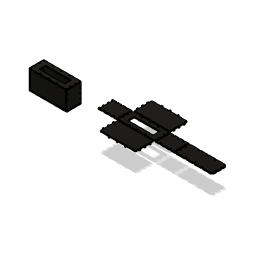
Case (Autodesk Fusion 360 design; units mm, degrees)
Autodesk Fusion 360 part; units mm, degrees
sketch "Sketch1" plane through (0, 0, 0) normal (0, 1, 0) x (1, 0, 0)
  line L0 (-40, -20) -> (150, -20)
  line L1 (150, -20) -> (150, 53.3)
  line L2 (150, 53.3) -> (-40, 53.3)
  line L3 (-40, 53.3) -> (-40, -20)
  line L4 (-40, 16.65) -> (-10, 16.65)
  line L5 (-10, -0.0029) -> (120, -0.0029)
  line L6 (120, 33.2971) -> (-10, 33.2971)
  line L7 (-10, 33.2971) -> (-10, -0.0029)
  line L8 (120, 33.2971) -> (120, -0.0029)
  dimension "d39" = 190
  dimension "d72" = 130
  dimension "d73" = 33.3
  constraint horizontal L0
  constraint vertical L1
  constraint horizontal L2
  constraint vertical L3
  constraint midpoint L3 L4.start
  constraint perpendicular L3 L4
  constraint vertical L7
  constraint perpendicular L5 L8
  measures "d39" distance of L1.end L2.end
  measures "d72" distance of L5.start L5.end
  measures "d73" distance of L5.start L6.end
extrude "Extrude6" add sketch "Sketch1" against normal blind 6 contours L0 L1 L2 L3 | L5 L6 L7 L8 makes body 1
sketch "Sketch3" plane through (-40, 0, 0) normal (-1, 0, 0) x (0, 0, 1)
  line L0 (20, 0) -> (-53.3, 0)
  line L1 (-53.3, 0) -> (-53.3, -6)
  line L2 (-53.3, -6) -> (20, -6)
  line L3 (20, -6) -> (20, 0)
  line L4 (-53.3, 0) -> (20, 0)
  line L5 (20, 0) -> (20, -100)
  line L6 (20, -100) -> (-53.3, -100)
  line L7 (-53.3, -100) -> (-53.3, 0)
  line L8 (20, 0) -> (14, 0)
  line L9 (14, 0) -> (14, -6)
  line L10 (20, -6) -> (20, 0)
  line L11 (14, -6) -> (-1, -6)
  line L12 (-7, -6) -> (-7, 0)
  line L13 (-7, 0) -> (-1, 0)
  line L14 (-1, 0) -> (-1, -6)
  line L15 (-53.3, 0) -> (-47.3, 0)
  line L16 (-47.3, 0) -> (-47.3, -6)
  line L17 (-53.3, -6) -> (-53.3, 0)
  line L18 (-47.3, -6) -> (-32.3, -6)
  line L19 (-26.3, -6) -> (-26.3, 0)
  line L20 (-26.3, 0) -> (-32.3, 0)
  line L21 (-32.3, 0) -> (-32.3, -6)
  dimension "d50" = 73.3
  dimension "d51" = 100
  dimension "d52" = 6
  dimension "d53" = 6
  dimension "d54" = 15
  dimension "d55" = 6
  dimension "d56" = 6
  dimension "d57" = 6
  dimension "d58" = 6
  dimension "d59" = 15
  dimension "d60" = 6
  dimension "d61" = 6
  constraint horizontal L4
  constraint vertical L5
  constraint horizontal L6
  constraint vertical L7
  constraint coincident L0.end L1.start
  constraint horizontal L8
  constraint vertical L9
  constraint vertical L10
  constraint coincident L0.start L3.end
  constraint perpendicular L9 L11
  constraint vertical L12
  constraint horizontal L13
  constraint vertical L14
  constraint horizontal L15
  constraint vertical L16
  constraint vertical L17
  constraint perpendicular L16 L18
  constraint vertical L19
  constraint horizontal L20
  constraint vertical L21
  measures "d50" distance of L0.end L0.start
  measures "d51" distance of L0.end L6.end
  measures "d52" distance of L0.start L8.end
  measures "d53" distance of L0.start L2.end
  measures "d54" distance of L9.end L11.end
  measures "d55" distance of L11.end L12.start
  measures "d56" distance of L11.end L13.end
  measures "d57" distance of L0.end L15.end
  measures "d58" distance of L0.end L1.end
  measures "d59" distance of L16.end L18.end
  measures "d60" distance of L18.end L19.start
  measures "d61" distance of L18.end L20.end
extrude "Extrude10" cut sketch "Sketch3" against normal blind 6 contours L0 L2 L3 L4 L5 L8 L9 L10 | L0 L2 L4 L12 L13 L14 | L0 L2 L4 L19 L20 L21 | L0 L1 L2 L4 L7 L15 L16 L17 bodies 1
extrude "Extrude7" cut sketch "Sketch3" against normal blind 6 contours L0 L1 L2 L4 L7 L15 L16 L17 bodies 1
extrude "Extrude8" cut sketch "Sketch3" against normal blind 6 contours L0 L2 L4 L19 L20 L21 bodies 1
extrude "Extrude9" cut sketch "Sketch3" against normal blind 6 contours L0 L2 L3 L4 L5 L8 L9 L10 | L0 L2 L4 L12 L13 L14 bodies 1
extrude "Extrude11" add sketch "Sketch3" against normal blind 6 separate body contours L0 L2 L3 L4 L5 L8 L9 L10 | L2 L5 L6 L7 L11 L18 | L0 L2 L4 L12 L13 L14 | L0 L2 L4 L19 L20 L21 | L0 L1 L2 L4 L7 L15 L16 L17 makes body 2
sketch "Sketch4" plane through (0, 0, 20) normal (0, 0, 1) x (1, 0, 0)
  line L0 (-40, 0) -> (-40, -100)
  line L1 (-40, -100) -> (-34, -100)
  line L2 (-34, -100) -> (-34, 0)
  line L3 (-34, 0) -> (-40, 0)
  line L4 (-40, 0) -> (150, 0)
  line L5 (150, 0) -> (150, -100)
  line L6 (150, -100) -> (-40, -100)
  line L7 (-40, -100) -> (-40, 0)
  line L8 (-40, 0) -> (-34, 0)
  line L9 (-34, 0) -> (-34, -6)
  line L10 (-34, -6) -> (-40, -6)
  line L11 (-40, -6) -> (-40, 0)
  line L12 (-40, -100) -> (-34, -100)
  line L13 (-34, -100) -> (-34, -94)
  line L14 (-34, -94) -> (-40, -94)
  line L15 (-40, -94) -> (-40, -100)
  line L16 (-40, -94) -> (-40, -79)
  line L17 (-40, -79) -> (-34, -79)
  line L18 (-34, -79) -> (-34, -73)
  line L19 (-34, -73) -> (-40, -73)
  line L20 (-40, -73) -> (-40, -79)
  line L21 (-40, -6) -> (-40, -21)
  line L22 (-40, -21) -> (-34, -21)
  line L23 (-34, -21) -> (-34, -27)
  line L24 (-34, -27) -> (-40, -27)
  line L25 (-40, -27) -> (-40, -21)
  line L26 (-40, -27) -> (-40, -47)
  line L27 (-40, -47) -> (-34, -47)
  line L28 (-34, -47) -> (-34, -53)
  line L29 (-34, -53) -> (-40, -53)
  line L30 (-40, -53) -> (-40, -47)
  line L31 (52, 0) -> (58, 0)
  line L32 (58, 0) -> (58, -6)
  line L33 (58, -6) -> (52, -6)
  line L34 (52, -6) -> (52, 0)
  line L35 (52, 0) -> (17, 0)
  line L36 (58, 0) -> (93, 0)
  line L37 (17, 0) -> (11, 0)
  line L38 (11, 0) -> (11, -6)
  line L39 (11, -6) -> (17, -6)
  line L40 (17, -6) -> (17, 0)
  line L41 (93, 0) -> (99, 0)
  line L42 (99, 0) -> (99, -6)
  line L43 (99, -6) -> (93, -6)
  line L44 (93, -6) -> (93, 0)
  line L45 (144, -27) -> (144, -21)
  line L46 (150, -27) -> (144, -27)
  line L47 (150, -53) -> (144, -53)
  line L48 (144, -73) -> (144, -79)
  line L49 (150, -79) -> (150, -73)
  line L50 (150, -73) -> (144, -73)
  line L51 (144, -79) -> (150, -79)
  line L52 (144, -47) -> (150, -47)
  line L53 (150, -47) -> (150, -53)
  line L54 (144, -27) -> (144, -47)
  line L55 (144, -53) -> (144, -47)
  line L56 (150, -21) -> (150, -27)
  line L57 (144, -21) -> (150, -21)
  line L58 (-34, -6) -> (150, -6)
  line L59 (150, 0) -> (144, 0)
  line L60 (144, 0) -> (144, -6)
  line L61 (144, -6) -> (150, -6)
  line L62 (150, -6) -> (150, 0)
  line L63 (144, -6) -> (144, -100)
  dimension "d76" = 6
  dimension "d77" = 6
  dimension "d78" = 6
  dimension "d79" = 6
  dimension "d80" = 15
  dimension "d81" = 6
  dimension "d82" = 6
  dimension "d83" = 15
  dimension "d84" = 6
  dimension "d85" = 6
  dimension "d86" = 20
  dimension "d87" = 6
  dimension "d88" = 6
  dimension "d93" = 190
  dimension "d95" = 6
  dimension "d96" = 6
  dimension "d97" = 35
  dimension "d98" = 35
  dimension "d99" = 6
  dimension "d100" = 6
  dimension "d101" = 6
  dimension "d102" = 6
  dimension "d103" = 6
  dimension "d104" = 6
  dimension "d105" = 6
  dimension "d106" = 6
  dimension "d107" = 20
  dimension "d108" = 6
  dimension "d109" = 6
  dimension "d122" = 6
  dimension "d123" = 6
  dimension "d124" = 94
  constraint horizontal L4
  constraint vertical L5
  constraint horizontal L6
  constraint vertical L7
  constraint coincident L0.start L3.end
  constraint horizontal L8
  constraint vertical L9
  constraint horizontal L10
  constraint vertical L11
  constraint horizontal L12
  constraint vertical L13
  constraint horizontal L14
  constraint vertical L15
  constraint coincident L0.end L1.start
  constraint perpendicular L14 L16
  constraint horizontal L17
  constraint vertical L18
  constraint horizontal L19
  constraint vertical L20
  constraint perpendicular L10 L21
  constraint horizontal L22
  constraint vertical L23
  constraint horizontal L24
  constraint vertical L25
  constraint perpendicular L24 L26
  constraint horizontal L27
  constraint vertical L28
  constraint horizontal L29
  constraint vertical L30
  constraint horizontal L31
  constraint vertical L32
  constraint horizontal L33
  constraint vertical L34
  constraint perpendicular L34 L35
  constraint perpendicular L32 L36
  constraint horizontal L37
  constraint vertical L38
  constraint horizontal L39
  constraint vertical L40
  constraint horizontal L41
  constraint vertical L42
  constraint horizontal L43
  constraint vertical L44
  constraint horizontal L51
  constraint vertical L49
  constraint horizontal L50
  constraint vertical L48
  constraint horizontal L57
  constraint vertical L56
  constraint horizontal L46
  constraint vertical L45
  constraint perpendicular L46 L54
  constraint horizontal L52
  constraint vertical L53
  constraint horizontal L47
  constraint vertical L55
  constraint coincident L5 L58.end
  constraint perpendicular L5 L58
  constraint horizontal L59
  constraint vertical L60
  constraint horizontal L61
  constraint vertical L62
  constraint perpendicular L46 L63
  measures "d76" distance of L0.start L2.end
  measures "d77" distance of L0.start L10.end
  measures "d78" distance of L0.end L1.end
  measures "d79" distance of L0.end L14.end
  measures "d80" distance of L14.end L16.end
  measures "d81" distance of L16.end L17.end
  measures "d82" distance of L16.end L19.end
  measures "d83" distance of L10.end L21.end
  measures "d84" distance of L21.end L22.end
  measures "d85" distance of L21.end L24.end
  measures "d86" distance of L24.end L26.end
  measures "d87" distance of L26.end L27.end
  measures "d88" distance of L26.end L29.end
  measures "d93" distance of L0.start L4.end
  measures "d95" distance of L31.start L31.end
  measures "d96" distance of L31.start L33.end
  measures "d97" distance of L31.start L35.end
  measures "d98" distance of L31.end L36.end
  measures "d99" distance of L35.end L37.end
  measures "d100" distance of L35.end L39.end
  measures "d101" distance of L36.end L41.end
  measures "d102" distance of L36.end L43.end
  measures "d103" distance of L49.start L48.end
  measures "d104" distance of L48.end L48.start
  measures "d105" distance of L56.start L45.end
  measures "d106" distance of L45.start L45.end
  measures "d107" distance of L45.start L52.start
  measures "d108" distance of L52.end L52.start
  measures "d109" distance of L47.end L52.start
  measures "d122" distance of L4.end L59.end
  measures "d123" distance of L4.end L58.end
  measures "d124" distance of L60.end L63.end
extrude "Extrude13" cut sketch "Sketch4" against normal blind 6 contours L0 L2 L7 L22 L23 L24 L25 | L0 L2 L7 L27 L28 L29 L30 | L0 L2 L7 L17 L18 L19 L20 bodies 2
extrude "Extrude12" cut sketch "Sketch1" against normal blind 6 contours L5 L6 L7 L8 bodies 1
copy_body "CopyPasteBodies1" bodies 2 makes body 3
move_body "Move1" bodies 3 to x (1, 0, 0) y (0, 1, 0) z (0, 0, 1) at (184, 0, 0)
sketch "Sketch5" plane through (0, 0, 0) normal (0, 1, 0) x (1, 0, 0)
  line L0 (150, 53.3) -> (144, 53.3)
  line L1 (144, 53.3) -> (144, 47.3)
  line L2 (144, 47.3) -> (150, 47.3)
  line L3 (150, 47.3) -> (150, 53.3)
  line L4 (150, 32.3) -> (144, 32.3)
  line L5 (144, 32.3) -> (144, 26.3)
  line L6 (144, 26.3) -> (150, 26.3)
  line L7 (150, 26.3) -> (150, 32.3)
  line L8 (150, 1) -> (144, 1)
  line L9 (144, 1) -> (144, 7)
  line L10 (144, 7) -> (150, 7)
  line L11 (150, 7) -> (150, 1)
  line L12 (150, -20) -> (144, -20)
  line L13 (144, -20) -> (144, -14)
  line L14 (144, -14) -> (150, -14)
  line L15 (150, -14) -> (150, -20)
  dimension "d110" = 6
  dimension "d111" = 6
  dimension "d112" = 6
  dimension "d113" = 6
  dimension "d114" = 6
  dimension "d115" = 6
  dimension "d116" = 6
  dimension "d117" = 6
  constraint horizontal L0
  constraint vertical L1
  constraint horizontal L2
  constraint vertical L3
  constraint horizontal L4
  constraint vertical L5
  constraint horizontal L6
  constraint vertical L7
  constraint horizontal L8
  constraint vertical L9
  constraint horizontal L10
  constraint vertical L11
  constraint horizontal L12
  constraint vertical L13
  constraint horizontal L14
  constraint vertical L15
  measures "d110" distance of L0.start L0.end
  measures "d111" distance of L0.start L2.end
  measures "d112" distance of L4.start L4.end
  measures "d113" distance of L4.start L6.end
  measures "d114" distance of L8.start L8.end
  measures "d115" distance of L8.start L10.end
  measures "d116" distance of L12.start L12.end
  measures "d117" distance of L12.start L14.end
extrude "Extrude15" cut sketch "Sketch5" against normal blind 6 bodies 1
extrude "Extrude16" cut sketch "Sketch4" against normal blind 6 contours L4 L37 L38 L39 L40 L58 | L4 L31 L32 L33 L34 L58 | L4 L41 L42 L43 L44 L58 bodies 1
extrude "Extrude17" add sketch "Sketch4" against normal blind 6 separate body contours L0 L2 L7 L22 L23 L24 L25 | L2 L6 L13 L18 L23 L28 L33 L39 L43 L45 L48 L54 L55 L58 L63 | L4 L37 L38 L39 L40 L58 | L0 L2 L7 L27 L28 L29 L30 | L4 L31 L32 L33 L34 L58 | L0 L2 L7 L17 L18 L19 L20 | L4 L41 L42 L43 L44 L58 | L5 L45 L46 L56 L57 L63 | L5 L48 L49 L50 L51 L63 | L5 L47 L52 L53 L55 L63 makes body 4
sketch "fundo" plane through (0, 0, -53.3) normal (0, 0, -1) x (-1, 0, 0)
  line L0 (40, -100) -> (40, 0)
  line L1 (40, 0) -> (34, 0)
  line L2 (34, 0) -> (34, -100)
  line L3 (34, -100) -> (40, -100)
  line L4 (40, 0) -> (-150, 0)
  line L5 (-150, 0) -> (-150, -100)
  line L6 (-150, -100) -> (40, -100)
  line L7 (40, -100) -> (40, 0)
  line L8 (-150, 0) -> (-144, 0)
  line L9 (-144, 0) -> (-144, -6)
  line L10 (-144, -6) -> (-150, -6)
  line L11 (-150, -6) -> (-150, 0)
  line L12 (-55, 0) -> (-58, 0)
  line L13 (-58, 0) -> (-52, 0)
  line L14 (-52, 0) -> (-52, -6)
  line L15 (-52, -6) -> (-58, -6)
  line L16 (-58, -6) -> (-58, 0)
  line L17 (-58, 0) -> (-93, 0)
  line L18 (-93, 0) -> (-99, 0)
  line L19 (-99, 0) -> (-99, -6)
  line L20 (-99, -6) -> (-93, -6)
  line L21 (-93, -6) -> (-93, 0)
  line L22 (-52, 0) -> (-17, 0)
  line L23 (-17, 0) -> (-11, 0)
  line L24 (-11, 0) -> (-11, -6)
  line L25 (-11, -6) -> (-17, -6)
  line L26 (-17, -6) -> (-17, 0)
  line L27 (-150, 0) -> (-150, -21)
  line L28 (40, 0) -> (40, -21)
  line L29 (-150, -21) -> (-144, -21)
  line L30 (-144, -21) -> (-144, -27)
  line L31 (-144, -27) -> (-150, -27)
  line L32 (-150, -27) -> (-150, -21)
  line L33 (40, -21) -> (34, -21)
  line L34 (34, -21) -> (34, -27)
  line L35 (34, -27) -> (40, -27)
  line L36 (40, -27) -> (40, -21)
  line L37 (-144, -27) -> (-144, -47)
  line L38 (-144, -47) -> (-150, -47)
  line L39 (-150, -47) -> (-150, -53)
  line L40 (-150, -53) -> (-144, -53)
  line L41 (-144, -53) -> (-144, -47)
  line L42 (-144, -53) -> (-144, -73)
  line L43 (-144, -73) -> (-150, -73)
  line L44 (-150, -73) -> (-150, -79)
  line L45 (-150, -79) -> (-144, -79)
  line L46 (-144, -79) -> (-144, -73)
  line L47 (40, -27) -> (40, -47)
  line L48 (40, -47) -> (34, -47)
  line L49 (34, -47) -> (34, -53)
  line L50 (34, -53) -> (40, -53)
  line L51 (40, -53) -> (40, -47)
  line L52 (40, -53) -> (40, -73)
  line L53 (40, -73) -> (34, -73)
  line L54 (34, -73) -> (34, -79)
  line L55 (34, -79) -> (40, -79)
  line L56 (40, -79) -> (40, -73)
  line L57 (34, 0) -> (34, -100)
  line L58 (-144, 0) -> (-144, -100)
  line L59 (-150, -6) -> (40, -6)
  dimension "d127" = 6
  dimension "d128" = 6
  dimension "d129" = 3
  dimension "d130" = 6
  dimension "d131" = 6
  dimension "d132" = 35
  dimension "d133" = 6
  dimension "d134" = 6
  dimension "d135" = 35
  dimension "d136" = 6
  dimension "d137" = 6
  dimension "d140" = 21
  dimension "d141" = 21
  dimension "d142" = 6
  dimension "d143" = 6
  dimension "d144" = 6
  dimension "d145" = 6
  dimension "d146" = 20
  dimension "d147" = 6
  dimension "d148" = 20
  dimension "d149" = 6
  dimension "d150" = 6
  dimension "d151" = 20
  dimension "d152" = 6
  dimension "d153" = 6
  dimension "d154" = 20
  dimension "d155" = 6
  dimension "d156" = 6
  dimension "d159" = 190
  constraint horizontal L4
  constraint vertical L5
  constraint horizontal L6
  constraint vertical L7
  constraint coincident L0.end L1.start
  constraint horizontal L8
  constraint vertical L9
  constraint horizontal L10
  constraint vertical L11
  constraint midpoint L4 L12.start
  constraint parallel L4 L12
  constraint horizontal L13
  constraint vertical L14
  constraint horizontal L15
  constraint vertical L16
  constraint perpendicular L16 L17
  constraint horizontal L18
  constraint vertical L19
  constraint horizontal L20
  constraint vertical L21
  constraint perpendicular L14 L22
  constraint horizontal L23
  constraint vertical L24
  constraint horizontal L25
  constraint vertical L26
  constraint perpendicular L4 L27
  constraint perpendicular L4 L28
  constraint horizontal L29
  constraint vertical L30
  constraint horizontal L31
  constraint vertical L32
  constraint horizontal L33
  constraint vertical L34
  constraint horizontal L35
  constraint vertical L36
  constraint perpendicular L31 L37
  constraint horizontal L38
  constraint vertical L39
  constraint horizontal L40
  constraint vertical L41
  constraint perpendicular L40 L42
  constraint horizontal L43
  constraint vertical L44
  constraint horizontal L45
  constraint vertical L46
  constraint perpendicular L35 L47
  constraint horizontal L48
  constraint vertical L49
  constraint horizontal L50
  constraint vertical L51
  constraint perpendicular L50 L52
  constraint horizontal L53
  constraint vertical L54
  constraint horizontal L55
  constraint vertical L56
  constraint coincident L1.end L2.start
  constraint coincident L2.end L3.start
  constraint coincident L6 L58.end
  constraint perpendicular L6 L58
  constraint horizontal L59
  measures "d127" distance of L4.end L8.end
  measures "d128" distance of L4.end L10.end
  measures "d129" distance of L12.start L12.end
  measures "d130" distance of L12.end L13.end
  measures "d131" distance of L12.end L15.end
  measures "d132" distance of L12.end L17.end
  measures "d133" distance of L17.end L18.end
  measures "d134" distance of L17.end L20.end
  measures "d135" distance of L13.end L22.end
  measures "d136" distance of L22.end L23.end
  measures "d137" distance of L22.end L25.end
  measures "d140" distance of L4.end L27.end
  measures "d141" distance of L0.end L28.end
  measures "d142" distance of L27.end L29.end
  measures "d143" distance of L27.end L31.end
  measures "d144" distance of L28.end L33.end
  measures "d145" distance of L28.end L35.end
  measures "d146" distance of L30.end L37.end
  measures "d147" distance of L37.end L40.end
  measures "d148" distance of L40.end L42.end
  measures "d149" distance of L42.end L43.end
  measures "d150" distance of L42.end L45.end
  measures "d151" distance of L35.end L47.end
  measures "d152" distance of L47.end L48.end
  measures "d153" distance of L47.end L50.end
  measures "d154" distance of L50.end L52.end
  measures "d155" distance of L52.end L53.end
  measures "d156" distance of L52.end L55.end
  measures "d159" distance of L10.end L59.end
extrude "Extrude18" cut sketch "fundo" against normal blind 6 contours L4 L23 L24 L25 L26 L59 | L4 L18 L19 L20 L21 L59 | L4 L12 L13 L14 L15 L16 L59 bodies 1
extrude "Extrude19" cut sketch "fundo" against normal blind 6 contours L0 L2 L7 L53 L54 L55 L56 L57 | L0 L2 L7 L48 L49 L50 L51 L57 | L5 L43 L44 L45 L46 L58 | L0 L2 L7 L33 L34 L35 L36 L57 | L5 L38 L39 L40 L41 L58 | L5 L29 L30 L31 L32 L58 bodies 2 3
extrude "Extrude20" add sketch "fundo" against normal blind 6 separate body contours L0 L2 L7 L53 L54 L55 L56 L57 | L2 L6 L15 L20 L25 L30 L34 L37 L41 L42 L46 L49 L54 L57 L58 L59 | L0 L2 L7 L48 L49 L50 L51 L57 | L5 L43 L44 L45 L46 L58 | L0 L2 L7 L33 L34 L35 L36 L57 | L5 L38 L39 L40 L41 L58 | L5 L29 L30 L31 L32 L58 | L4 L23 L24 L25 L26 L59 | L4 L18 L19 L20 L21 L59 | L4 L12 L13 L14 L15 L16 L59 makes body 5
sketch "Sketch7" plane through (0, -100, 0) normal (0, -1, 0) x (1, 0, 0)
  line L0 (-34, -53.3) -> (144, -53.3)
  line L1 (144, -53.3) -> (144, -47.3)
  line L2 (144, -47.3) -> (-34, -47.3)
  line L3 (-34, -47.3) -> (-34, -53.3)
  line L4 (-40, -53.3) -> (150, -53.3)
  line L5 (150, -53.3) -> (150, 20)
  line L6 (150, 20) -> (-40, 20)
  line L7 (-40, 20) -> (-40, -53.3)
  line L8 (144, -53.3) -> (150, -53.3)
  line L9 (150, -53.3) -> (150, 20)
  line L10 (150, 20) -> (144, 20)
  line L11 (144, 20) -> (144, -53.3)
  line L12 (-34, -53.3) -> (-40, -53.3)
  line L13 (-40, -53.3) -> (-40, 20)
  line L14 (-40, 20) -> (-34, 20)
  line L15 (-34, 20) -> (-34, -53.3)
  line L16 (-40, 20) -> (150, 20)
  line L17 (150, 20) -> (150, 14)
  line L18 (150, 14) -> (-40, 14)
  line L19 (-40, 14) -> (-40, 20)
  line L20 (55, 14) -> (52.5, 14)
  line L21 (52.5, 14) -> (57.5, 14)
  arc A0 (52.5, 14) -> (57.5, 14) centre (55, 12.125) ccw
  line L22 (-40, 14) -> (-40, -1)
  line L23 (-40, -1) -> (-34, -1)
  line L24 (-34, -1) -> (-34, -7)
  line L25 (-34, -7) -> (-40, -7)
  line L26 (-40, -7) -> (-40, -1)
  line L27 (-40, -7) -> (-40, -26.3)
  line L28 (-40, -26.3) -> (-34, -26.3)
  line L29 (-34, -26.3) -> (-34, -32.3)
  line L30 (-34, -32.3) -> (-40, -32.3)
  line L31 (-40, -32.3) -> (-40, -26.3)
  line L32 (-40, -53.3) -> (-34, -53.3)
  line L33 (-34, -53.3) -> (-34, -47.3)
  line L34 (-34, -47.3) -> (-40, -47.3)
  line L35 (-40, -47.3) -> (-40, -53.3)
  line L36 (150, -47.3) -> (150, -53.3)
  line L37 (150, -7) -> (144, -7)
  line L38 (144, -1) -> (150, -1)
  line L39 (144, -26.3) -> (150, -26.3)
  line L40 (144, -47.3) -> (144, -53.3)
  line L41 (144, -53.3) -> (144, 20)
  line L42 (144, 14) -> (144, -1)
  line L43 (144, 14) -> (144, 20)
  line L44 (150, -32.3) -> (144, -32.3)
  line L45 (150, -47.3) -> (144, -47.3)
  line L46 (144, -53.3) -> (150, -53.3)
  line L47 (150, -53.3) -> (150, -47.3)
  line L48 (144, 20) -> (150, 20)
  line L49 (150, -1) -> (150, -7)
  line L50 (144, -7) -> (144, -1)
  line L51 (150, -53.3) -> (144, -53.3)
  line L52 (150, -26.3) -> (150, -32.3)
  line L53 (144, -7) -> (144, -26.3)
  line L54 (150, 20) -> (150, -53.3)
  line L55 (144, 20) -> (144, -53.3)
  line L56 (144, -32.3) -> (144, -26.3)
  line L57 (-34, 20) -> (11, 20)
  line L58 (11, 20) -> (11, 14)
  line L59 (11, 14) -> (-34, 14)
  line L60 (-34, 14) -> (-34, 20)
  line L61 (11, 20) -> (17, 20)
  line L62 (17, 20) -> (17, 14)
  line L63 (17, 14) -> (11, 14)
  line L64 (11, 14) -> (11, 20)
  line L65 (17, 20) -> (52, 20)
  line L66 (52, 20) -> (52, 14)
  line L67 (52, 14) -> (17, 14)
  line L68 (17, 14) -> (17, 20)
  line L69 (52, 20) -> (58, 20)
  line L70 (58, 20) -> (58, 14)
  line L71 (58, 14) -> (52, 14)
  line L72 (52, 14) -> (52, 20)
  line L73 (58, 20) -> (93, 20)
  line L74 (93, 20) -> (93, 14)
  line L75 (93, 14) -> (58, 14)
  line L76 (58, 14) -> (58, 20)
  line L77 (93, 20) -> (99, 20)
  line L78 (99, 20) -> (99, 14)
  line L79 (99, 14) -> (93, 14)
  line L80 (93, 14) -> (93, 20)
  line L81 (144, -53.3) -> (99, -53.3)
  line L82 (99, -53.3) -> (93, -53.3)
  line L83 (93, -53.3) -> (93, -47.3)
  line L84 (93, -47.3) -> (99, -47.3)
  line L85 (99, -47.3) -> (99, -53.3)
  line L86 (93, -53.3) -> (58, -53.3)
  line L87 (58, -53.3) -> (58, -47.3)
  line L88 (58, -47.3) -> (93, -47.3)
  line L89 (93, -47.3) -> (93, -53.3)
  line L90 (58, -53.3) -> (52, -53.3)
  line L91 (52, -53.3) -> (52, -47.3)
  line L92 (52, -47.3) -> (58, -47.3)
  line L93 (58, -47.3) -> (58, -53.3)
  line L94 (52, -53.3) -> (17, -53.3)
  line L95 (17, -53.3) -> (17, -47.3)
  line L96 (17, -47.3) -> (52, -47.3)
  line L97 (52, -47.3) -> (52, -53.3)
  line L98 (17, -53.3) -> (11, -53.3)
  line L99 (11, -53.3) -> (11, -47.3)
  line L100 (11, -47.3) -> (17, -47.3)
  line L101 (17, -47.3) -> (17, -53.3)
  dimension "d162" = 190
  dimension "d163" = 73.3
  dimension "d164" = 6
  dimension "d169" = 5
  dimension "d171" = 3.125
  dimension "d172" = 15
  dimension "d173" = 6
  dimension "d174" = 6
  dimension "d175" = 19.3
  dimension "d176" = 6
  dimension "d177" = 6
  dimension "d178" = 6
  dimension "d179" = 6
  dimension "d182" = 73.3
  dimension "d183" = 6
  dimension "d184" = 15
  dimension "d185" = 6
  dimension "d186" = 6
  dimension "d187" = 19.3
  dimension "d188" = 6
  dimension "d189" = 6
  dimension "d190" = 6
  dimension "d191" = 6
  dimension "d194" = 45
  dimension "d195" = 6
  dimension "d196" = 6
  dimension "d197" = 6
  dimension "d198" = 35
  dimension "d199" = 6
  dimension "d200" = 6
  dimension "d201" = 6
  dimension "d202" = 35
  dimension "d203" = 6
  dimension "d204" = 6
  dimension "d205" = 6
  dimension "d208" = 45
  dimension "d209" = 6
  dimension "d210" = 6
  dimension "d211" = 35
  dimension "d212" = 6
  dimension "d213" = 6
  dimension "d214" = 6
  dimension "d215" = 35
  dimension "d216" = 6
  dimension "d217" = 6
  dimension "d218" = 6
  constraint horizontal L4
  constraint vertical L5
  constraint horizontal L6
  constraint vertical L7
  constraint horizontal L8
  constraint vertical L9
  constraint horizontal L10
  constraint vertical L11
  constraint coincident L0.end L1.start
  constraint horizontal L12
  constraint vertical L13
  constraint horizontal L14
  constraint vertical L15
  constraint coincident L0.start L3.end
  constraint horizontal L16
  constraint vertical L17
  constraint horizontal L18
  constraint vertical L19
  constraint symmetric L18 L20.end L21.start
  constraint symmetric L18 L21.end A0.end
  constraint perpendicular L18 L22
  constraint horizontal L23
  constraint vertical L24
  constraint horizontal L25
  constraint vertical L26
  constraint perpendicular L25 L27
  constraint horizontal L28
  constraint vertical L29
  constraint horizontal L30
  constraint vertical L31
  constraint horizontal L32
  constraint vertical L33
  constraint horizontal L34
  constraint vertical L35
  constraint vertical L55
  constraint horizontal L51
  constraint vertical L41
  constraint horizontal L48
  constraint vertical L54
  constraint coincident L4.end L5.start
  constraint vertical L43
  constraint horizontal L38
  constraint vertical L49
  constraint horizontal L37
  constraint vertical L50
  constraint perpendicular L37 L53
  constraint horizontal L39
  constraint vertical L52
  constraint horizontal L44
  constraint vertical L56
  constraint horizontal L46
  constraint vertical L47
  constraint horizontal L45
  constraint vertical L40
  constraint horizontal L57
  constraint vertical L58
  constraint horizontal L59
  constraint vertical L60
  constraint horizontal L61
  constraint vertical L62
  constraint horizontal L63
  constraint vertical L64
  constraint horizontal L65
  constraint vertical L66
  constraint horizontal L67
  constraint vertical L68
  constraint horizontal L69
  constraint vertical L70
  constraint horizontal L71
  constraint vertical L72
  constraint horizontal L73
  constraint vertical L74
  constraint horizontal L75
  constraint vertical L76
  constraint horizontal L77
  constraint vertical L78
  constraint horizontal L79
  constraint vertical L80
  constraint perpendicular L11 L81
  constraint horizontal L82
  constraint vertical L83
  constraint horizontal L84
  constraint vertical L85
  constraint horizontal L86
  constraint vertical L87
  constraint horizontal L88
  constraint vertical L89
  constraint horizontal L90
  constraint vertical L91
  constraint horizontal L92
  constraint vertical L93
  constraint horizontal L94
  constraint vertical L95
  constraint horizontal L96
  constraint vertical L97
  constraint horizontal L98
  constraint vertical L99
  constraint horizontal L100
  constraint vertical L101
  measures "d162" distance of L4.start L4.end
  measures "d163" distance of L4.start L6.end
  measures "d164" distance of L6.end L18.end
  measures "d169" distance of L20.end L21.end
  measures "d171" radius of A0
  measures "d172" distance of L18.end L22.end
  measures "d173" distance of L22.end L23.end
  measures "d174" distance of L22.end L25.end
  measures "d175" distance of L25.end L27.end
  measures "d176" distance of L27.end L28.end
  measures "d177" distance of L27.end L30.end
  measures "d178" distance of L4.start L0.start
  measures "d179" distance of L4.start L34.end
  measures "d182" distance of L0.end L10.end
  measures "d183" distance of L10.end L42.start
  measures "d184" distance of L38.start L42.start
  measures "d185" distance of L38.start L38.end
  measures "d186" distance of L38.start L37.end
  measures "d187" distance of L39.start L37.end
  measures "d188" distance of L39.end L39.start
  measures "d189" distance of L39.start L44.end
  measures "d190" distance of L4.end L0.end
  measures "d191" distance of L1.end L0.end
  measures "d194" distance of L14.end L57.end
  measures "d195" distance of L14.end L59.end
  measures "d196" distance of L57.end L61.end
  measures "d197" distance of L57.end L58.end
  measures "d198" distance of L61.end L65.end
  measures "d199" distance of L61.end L62.end
  measures "d200" distance of L65.end L69.end
  measures "d201" distance of L65.end L66.end
  measures "d202" distance of L69.end L73.end
  measures "d203" distance of L69.end L70.end
  measures "d204" distance of L73.end L77.end
  measures "d205" distance of L73.end L74.end
  measures "d208" distance of L0.end L81.end
  measures "d209" distance of L81.end L82.end
  measures "d210" distance of L81.end L84.end
  measures "d211" distance of L82.end L86.end
  measures "d212" distance of L82.end L83.end
  measures "d213" distance of L86.end L90.end
  measures "d214" distance of L86.end L87.end
  measures "d215" distance of L90.end L94.end
  measures "d216" distance of L90.end L91.end
  measures "d217" distance of L94.end L98.end
  measures "d218" distance of L94.end L95.end
extrude "Extrude23" cut sketch "Sketch7" against normal blind 6 contours L6 L15 L16 L18 L57 L58 L59 L60 L64 | L6 L16 L18 L62 L65 L66 L67 L68 L72 | L6 L16 L18 L70 L73 L74 L75 L76 L80 | L6 L11 L16 L18 L41 L43 L55 L78 bodies 4
extrude "Extrude22" cut sketch "Sketch7" against normal blind 6 contours L5 L9 L11 L41 L44 L45 L54 L55 | L5 L9 L11 L37 L39 L41 L53 L54 L55 | L5 L9 L11 L18 L38 L41 L42 L54 L55 bodies 3
extrude "Extrude21" cut sketch "Sketch7" against normal blind 6 contours L7 L13 L15 L30 L34 | L7 L13 L15 L25 L27 L28 | L7 L13 L15 L18 L22 L23 bodies 2
extrude "Extrude24" cut sketch "Sketch7" against normal blind 6 contours L0 L2 L3 L4 L15 L33 L99 | L0 L2 L4 L91 L94 L95 L96 L97 L101 | L0 L2 L4 L83 L86 L87 L88 L89 L93 | L0 L1 L2 L4 L11 L40 L41 L55 L81 L85 bodies 5
extrude "Extrude25" add sketch "Sketch7" against normal blind 6 separate body contours L0 L2 L3 L4 L15 L33 L99 | L2 L11 L15 L18 A0 L24 L29 L41 L42 L50 L53 L55 L56 L59 L63 L67 L71 L75 L79 L84 L88 L92 L96 L100 | L7 L13 L15 L30 L34 | L0 L2 L4 L91 L94 L95 L96 L97 L101 | L7 L13 L15 L25 L27 L28 | L0 L2 L4 L83 L86 L87 L88 L89 L93 | L7 L13 L15 L18 L22 L23 | L0 L1 L2 L4 L11 L40 L41 L55 L81 L85 | L6 L15 L16 L18 L57 L58 L59 L60 L64 | L5 L9 L11 L41 L44 L45 L54 L55 | L6 L16 L18 L62 L65 L66 L67 L68 L72 | L5 L9 L11 L37 L39 L41 L53 L54 L55 | L6 L16 L18 L70 L73 L74 L75 L76 L80 | L5 L9 L11 L18 L38 L41 L42 L54 L55 | L6 L11 L16 L18 L41 L43 L55 L78 makes body 6
copy_body "CopyPasteBodies2" bodies 1 6 2 5 3 4 makes body 7 makes body 8 makes body 9 makes body 10 makes body 11 makes body 12
move_body "Move2" bodies 7 8 9 10 11 12 to x (1, 0, 0) y (0, 1, 0) z (0, 0, 1) at (250, 0, 0)
move_body "Move3" bodies 10 to x (1, 0, 0) y (0, 0, 1) z (0, -1, 0) at (0, -53.3, -53.3)
move_body "Move4" bodies 12 to x (1, 0, 0) y (0, 0, -1) z (0, 1, 0) at (0, -20, 20)
move_body "Move5" bodies 12 10 7 9 8 11 to x (1, 0, 0) y (0, 1, 0) z (0, 0, 1) at (200, 0, 0)
move_body "Move6" bodies 9 to x (0, -1, 0) y (1, 0, 0) z (0, 0, 1) at (410, 410, 0)
move_body "Move7" bodies 8 to x (0, 1, 0) y (-1, 0, 0) z (0, 0, 1) at (500, -700, 0)
move_body "Move8" bodies 8 11 to x (0, 1, 0) y (-1, 0, 0) z (0, 0, 1) at (600, -600, 0)
sketch "cima plano" plane through (0, 0, 0) normal (0, 1, 0) x (-1, 0, 0)
  line L0 (-502, -153.3) -> (-502, -147.3)
  line L1 (-502, -147.3) -> (-467, -147.3)
  line L2 (-467, -147.3) -> (-467, -153.3)
  line L3 (-467, -153.3) -> (-461, -153.3)
  line L4 (-461, -153.3) -> (-461, -147.3)
  line L5 (-461, -147.3) -> (-416, -147.3)
  line L6 (-416, -147.3) -> (-416, -132.3)
  line L7 (-416, -132.3) -> (-410, -132.3)
  line L8 (-410, -132.3) -> (-410, -126.3)
  line L9 (-410, -126.3) -> (-416, -126.3)
  line L10 (-416, -126.3) -> (-416, -106.3)
  line L11 (-416, -106.3) -> (-410, -106.3)
  line L12 (-410, -106.3) -> (-410, -100.3)
  line L13 (-410, -100.3) -> (-416, -100.3)
  line L14 (-416, -100.3) -> (-416, -80.3)
  line L15 (-416, -80.3) -> (-410, -80.3)
  line L16 (-410, -80.3) -> (-410, -74.3)
  line L17 (-410, -74.3) -> (-416, -74.3)
  line L18 (-416, -74.3) -> (-416, -59.3)
  line L19 (-416, -59.3) -> (-461, -59.3)
  line L20 (-461, -59.3) -> (-461, -53.3)
  line L21 (-461, -53.3) -> (-467, -53.3)
  line L22 (-467, -53.3) -> (-467, -59.3)
  line L23 (-467, -59.3) -> (-502, -59.3)
  line L24 (-502, -59.3) -> (-502, -53.3)
  line L25 (-502, -53.3) -> (-508, -53.3)
  line L26 (-508, -53.3) -> (-508, -59.3)
  line L27 (-508, -59.3) -> (-543, -59.3)
  line L28 (-543, -59.3) -> (-543, -53.3)
  line L29 (-543, -53.3) -> (-549, -53.3)
  line L30 (-549, -53.3) -> (-549, -59.3)
  line L31 (-549, -59.3) -> (-594, -59.3)
  line L32 (-594, -59.3) -> (-594, -74.3)
  line L33 (-594, -74.3) -> (-600, -74.3)
  line L34 (-600, -74.3) -> (-600, -80.3)
  line L35 (-600, -80.3) -> (-594, -80.3)
  line L36 (-594, -80.3) -> (-594, -100.3)
  line L37 (-594, -100.3) -> (-600, -100.3)
  line L38 (-600, -100.3) -> (-600, -106.3)
  line L39 (-600, -106.3) -> (-594, -106.3)
  line L40 (-594, -106.3) -> (-594, -126.3)
  line L41 (-594, -126.3) -> (-600, -126.3)
  line L42 (-600, -126.3) -> (-600, -132.3)
  line L43 (-600, -132.3) -> (-594, -132.3)
  line L44 (-594, -132.3) -> (-594, -147.3)
  line L45 (-594, -147.3) -> (-549, -147.3)
  line L46 (-549, -147.3) -> (-549, -153.3)
  line L47 (-549, -153.3) -> (-543, -153.3)
  line L48 (-543, -153.3) -> (-543, -147.3)
  line L49 (-543, -147.3) -> (-508, -147.3)
  line L50 (-508, -147.3) -> (-508, -153.3)
  line L51 (-508, -153.3) -> (-502, -153.3)
  dimension "d232" = 45
  dimension "d233" = 35
  dimension "d234" = 35
  dimension "d236" = 45
  dimension "d237" = 178
  dimension "d238" = 15
  dimension "d239" = 20
  dimension "d240" = 6
  dimension "d241" = 6
  dimension "d242" = 20
  dimension "d243" = 15
  dimension "d244" = 88
  dimension "d247" = 190
  dimension "d250" = 6
  dimension "d257" = 100
  measures "d232" distance of L4.end L5.end
  measures "d233" distance of L0.end L1.end
  measures "d234" distance of L48.end L49.end
  measures "d236" distance of L44.end L45.end
  measures "d237" distance of L6 L44
  measures "d238" distance of L5.end L6.end
  measures "d239" distance of L9.end L10.end
  measures "d240" distance of L7.end L8.end
  measures "d241" distance of L6.end L7.end
  measures "d242" distance of L13.end L14.end
  measures "d243" distance of L17.end L18.end
  measures "d244" distance of L5 L19
  measures "d247" distance of L16 L34
  measures "d250" distance of L23.end L24.end
  measures "d257" distance of L3 L21
sketch "esquerda plano" plane through (0, 0, 0) normal (0, 1, 0) x (-1, 0, 0)
  line L0 (-316, -32.3) -> (-310, -32.3)
  line L1 (-310, -32.3) -> (-310, -26.3)
  line L2 (-310, -26.3) -> (-316, -26.3)
  line L3 (-316, -26.3) -> (-316, -7)
  line L4 (-316, -7) -> (-310, -7)
  line L5 (-310, -7) -> (-310, -1)
  line L6 (-310, -1) -> (-316, -1)
  line L7 (-316, -1) -> (-316, 14)
  line L8 (-316, 14) -> (-310, 14)
  line L9 (-310, 14) -> (-310, 20)
  line L10 (-310, 20) -> (-331, 20)
  line L11 (-331, 20) -> (-331, 14)
  line L12 (-331, 14) -> (-337, 14)
  line L13 (-337, 14) -> (-337, 20)
  line L14 (-337, 20) -> (-357, 20)
  line L15 (-357, 20) -> (-357, 14)
  line L16 (-357, 14) -> (-363, 14)
  line L17 (-363, 14) -> (-363, 20)
  line L18 (-363, 20) -> (-383, 20)
  line L19 (-383, 20) -> (-383, 14)
  line L20 (-383, 14) -> (-389, 14)
  line L21 (-389, 14) -> (-389, 20)
  line L22 (-389, 20) -> (-410, 20)
  line L23 (-410, 20) -> (-410, 14)
  line L24 (-410, 14) -> (-404, 14)
  line L25 (-404, 14) -> (-404, -1)
  line L26 (-404, -1) -> (-410, -1)
  line L27 (-410, -1) -> (-410, -7)
  line L28 (-410, -7) -> (-404, -7)
  line L29 (-404, -7) -> (-404, -26.3)
  line L30 (-404, -26.3) -> (-410, -26.3)
  line L31 (-410, -26.3) -> (-410, -32.3)
  line L32 (-410, -32.3) -> (-404, -32.3)
  line L33 (-404, -32.3) -> (-404, -47.3)
  line L34 (-404, -47.3) -> (-410, -47.3)
  line L35 (-410, -47.3) -> (-410, -53.3)
  line L36 (-410, -53.3) -> (-389, -53.3)
  line L37 (-389, -53.3) -> (-389, -47.3)
  line L38 (-389, -47.3) -> (-383, -47.3)
  line L39 (-383, -47.3) -> (-383, -53.3)
  line L40 (-383, -53.3) -> (-363, -53.3)
  line L41 (-363, -53.3) -> (-363, -47.3)
  line L42 (-363, -47.3) -> (-357, -47.3)
  line L43 (-357, -47.3) -> (-357, -53.3)
  line L44 (-357, -53.3) -> (-337, -53.3)
  line L45 (-337, -53.3) -> (-337, -47.3)
  line L46 (-337, -47.3) -> (-331, -47.3)
  line L47 (-331, -47.3) -> (-331, -53.3)
  line L48 (-331, -53.3) -> (-310, -53.3)
  line L49 (-310, -53.3) -> (-310, -47.3)
  line L50 (-310, -47.3) -> (-316, -47.3)
  line L51 (-316, -47.3) -> (-316, -32.3)
sketch "frente plano" plane through (0, 0, 0) normal (0, 1, 0) x (-1, 0, 0)
  line L0 (-543, -47.3) -> (-543, -53.3)
  line L1 (-543, -53.3) -> (-508, -53.3)
  line L2 (-508, -53.3) -> (-508, -47.3)
  line L3 (-508, -47.3) -> (-502, -47.3)
  line L4 (-502, -47.3) -> (-502, -53.3)
  line L5 (-502, -53.3) -> (-467, -53.3)
  line L6 (-467, -53.3) -> (-467, -47.3)
  line L7 (-467, -47.3) -> (-461, -47.3)
  line L8 (-461, -47.3) -> (-461, -53.3)
  line L9 (-461, -53.3) -> (-416, -53.3)
  line L10 (-416, -53.3) -> (-416, -47.3)
  line L11 (-416, -47.3) -> (-410, -47.3)
  line L12 (-410, -47.3) -> (-410, -32.3)
  line L13 (-410, -32.3) -> (-416, -32.3)
  line L14 (-416, -32.3) -> (-416, -26.3)
  line L15 (-416, -26.3) -> (-410, -26.3)
  line L16 (-410, -26.3) -> (-410, -7)
  line L17 (-410, -7) -> (-416, -7)
  line L18 (-416, -7) -> (-416, -1)
  line L19 (-416, -1) -> (-410, -1)
  line L20 (-410, -1) -> (-410, 14)
  line L21 (-410, 14) -> (-416, 14)
  line L22 (-416, 14) -> (-416, 20)
  line L23 (-416, 20) -> (-461, 20)
  line L24 (-461, 20) -> (-461, 14)
  line L25 (-461, 14) -> (-467, 14)
  line L26 (-467, 14) -> (-467, 20)
  line L27 (-467, 20) -> (-502, 20)
  line L28 (-502, 20) -> (-502, 14)
  line L29 (-502, 14) -> (-508, 14)
  line L30 (-508, 14) -> (-508, 20)
  line L31 (-508, 20) -> (-543, 20)
  line L32 (-543, 20) -> (-543, 14)
  line L33 (-543, 14) -> (-549, 14)
  line L34 (-549, 14) -> (-549, 20)
  line L35 (-549, 20) -> (-594, 20)
  line L36 (-594, 20) -> (-594, 14)
  line L37 (-594, 14) -> (-600, 14)
  line L38 (-600, 14) -> (-600, -1)
  line L39 (-600, -1) -> (-594, -1)
  line L40 (-594, -1) -> (-594, -7)
  line L41 (-594, -7) -> (-600, -7)
  line L42 (-600, -7) -> (-600, -26.3)
  line L43 (-600, -26.3) -> (-594, -26.3)
  line L44 (-594, -26.3) -> (-594, -32.3)
  line L45 (-594, -32.3) -> (-600, -32.3)
  line L46 (-600, -32.3) -> (-600, -47.3)
  line L47 (-600, -47.3) -> (-594, -47.3)
  line L48 (-594, -47.3) -> (-594, -53.3)
  line L49 (-594, -53.3) -> (-549, -53.3)
  line L50 (-549, -53.3) -> (-549, -47.3)
  line L51 (-549, -47.3) -> (-543, -47.3)
  line L52 (-570, 0.0029) -> (-440, 0.0029)
  line L53 (-440, 0.0029) -> (-440, -33.2971)
  line L54 (-440, -33.2971) -> (-570, -33.2971)
  line L55 (-570, -33.2971) -> (-570, 0.0029)
  line L56 (-890, -47.3) -> (-890, -32.3)
  line L57 (40, -53.3) -> (40, 20)
  line L58 (-467, 120) -> (-461, 120)
  line L59 (-467, -153.3) -> (-461, -153.3)
  dimension "d258" = 930
  dimension "d259" = 273.3
  measures "d258" distance of L56 L57
  measures "d259" distance of L58 L59
sketch "direita plano" plane through (0, 0, 0) normal (0, 1, 0) x (-1, 0, 0)
  line L0 (-694, -1) -> (-700, -1)
  line L1 (-700, -1) -> (-700, -7)
  line L2 (-700, -7) -> (-694, -7)
  line L3 (-694, -7) -> (-694, -26.3)
  line L4 (-694, -26.3) -> (-700, -26.3)
  line L5 (-700, -26.3) -> (-700, -32.3)
  line L6 (-700, -32.3) -> (-694, -32.3)
  line L7 (-694, -32.3) -> (-694, -47.3)
  line L8 (-694, -47.3) -> (-700, -47.3)
  line L9 (-700, -47.3) -> (-700, -53.3)
  line L10 (-700, -53.3) -> (-679, -53.3)
  line L11 (-679, -53.3) -> (-679, -47.3)
  line L12 (-679, -47.3) -> (-673, -47.3)
  line L13 (-673, -47.3) -> (-673, -53.3)
  line L14 (-673, -53.3) -> (-653, -53.3)
  line L15 (-653, -53.3) -> (-653, -47.3)
  line L16 (-653, -47.3) -> (-647, -47.3)
  line L17 (-647, -47.3) -> (-647, -53.3)
  line L18 (-647, -53.3) -> (-627, -53.3)
  line L19 (-627, -53.3) -> (-627, -47.3)
  line L20 (-627, -47.3) -> (-621, -47.3)
  line L21 (-621, -47.3) -> (-621, -53.3)
  line L22 (-621, -53.3) -> (-600, -53.3)
  line L23 (-600, -53.3) -> (-600, -47.3)
  line L24 (-600, -47.3) -> (-606, -47.3)
  line L25 (-606, -47.3) -> (-606, -32.3)
  line L26 (-606, -32.3) -> (-600, -32.3)
  line L27 (-600, -32.3) -> (-600, -26.3)
  line L28 (-600, -26.3) -> (-606, -26.3)
  line L29 (-606, -26.3) -> (-606, -7)
  line L30 (-606, -7) -> (-600, -7)
  line L31 (-600, -7) -> (-600, -1)
  line L32 (-600, -1) -> (-606, -1)
  line L33 (-606, -1) -> (-606, 14)
  line L34 (-606, 14) -> (-600, 14)
  line L35 (-600, 14) -> (-600, 20)
  line L36 (-600, 20) -> (-621, 20)
  line L37 (-621, 20) -> (-621, 14)
  line L38 (-621, 14) -> (-627, 14)
  line L39 (-627, 14) -> (-627, 20)
  line L40 (-627, 20) -> (-647, 20)
  line L41 (-647, 20) -> (-647, 14)
  line L42 (-647, 14) -> (-653, 14)
  line L43 (-653, 14) -> (-653, 20)
  line L44 (-653, 20) -> (-673, 20)
  line L45 (-673, 20) -> (-673, 14)
  line L46 (-673, 14) -> (-679, 14)
  line L47 (-679, 14) -> (-679, 20)
  line L48 (-679, 20) -> (-700, 20)
  line L49 (-700, 20) -> (-700, 14)
  line L50 (-700, 14) -> (-694, 14)
  line L51 (-694, 14) -> (-694, -1)
sketch "traseira plano" plane through (0, 0, 0) normal (0, 1, 0) x (-1, 0, 0)
  line L0 (-884, -53.3) -> (-839, -53.3)
  line L1 (-839, -53.3) -> (-839, -47.3)
  line L2 (-839, -47.3) -> (-833, -47.3)
  line L3 (-833, -47.3) -> (-833, -53.3)
  line L4 (-833, -53.3) -> (-798, -53.3)
  line L5 (-798, -53.3) -> (-798, -47.3)
  line L6 (-798, -47.3) -> (-792, -47.3)
  line L7 (-792, -47.3) -> (-792, -53.3)
  line L8 (-792, -53.3) -> (-757, -53.3)
  line L9 (-757, -53.3) -> (-757, -47.3)
  line L10 (-757, -47.3) -> (-751, -47.3)
  line L11 (-751, -47.3) -> (-751, -53.3)
  line L12 (-751, -53.3) -> (-706, -53.3)
  line L13 (-706, -53.3) -> (-706, -47.3)
  line L14 (-706, -47.3) -> (-700, -47.3)
  line L15 (-700, -47.3) -> (-700, -32.3)
  line L16 (-700, -32.3) -> (-706, -32.3)
  line L17 (-706, -32.3) -> (-706, -26.3)
  line L18 (-706, -26.3) -> (-700, -26.3)
  line L19 (-700, -26.3) -> (-700, -7)
  line L20 (-700, -7) -> (-706, -7)
  line L21 (-706, -7) -> (-706, -1)
  line L22 (-706, -1) -> (-700, -1)
  line L23 (-700, -1) -> (-700, 14)
  line L24 (-700, 14) -> (-706, 14)
  line L25 (-706, 14) -> (-706, 20)
  line L26 (-706, 20) -> (-751, 20)
  line L27 (-751, 20) -> (-751, 14)
  line L28 (-751, 14) -> (-757, 14)
  line L29 (-757, 14) -> (-757, 20)
  line L30 (-757, 20) -> (-792, 20)
  line L31 (-792, 20) -> (-792, 14)
  line L32 (-792, 14) -> (-792.5, 14)
  arc A0 (-797.5, 14) -> (-792.5, 14) centre (-795, 12.125) ccw
  line L33 (-797.5, 14) -> (-798, 14)
  line L34 (-798, 14) -> (-798, 20)
  line L35 (-798, 20) -> (-833, 20)
  line L36 (-833, 20) -> (-833, 14)
  line L37 (-833, 14) -> (-839, 14)
  line L38 (-839, 14) -> (-839, 20)
  line L39 (-839, 20) -> (-884, 20)
  line L40 (-884, 20) -> (-884, 14)
  line L41 (-884, 14) -> (-890, 14)
  line L42 (-890, 14) -> (-890, -1)
  line L43 (-890, -1) -> (-884, -1)
  line L44 (-884, -1) -> (-884, -7)
  line L45 (-884, -7) -> (-890, -7)
  line L46 (-890, -7) -> (-890, -26.3)
  line L47 (-890, -26.3) -> (-884, -26.3)
  line L48 (-884, -26.3) -> (-884, -32.3)
  line L49 (-884, -32.3) -> (-890, -32.3)
  line L50 (-890, -32.3) -> (-890, -47.3)
  line L51 (-890, -47.3) -> (-884, -47.3)
  line L52 (-884, -47.3) -> (-884, -53.3)
sketch "fundo plano" plane through (0, 0, 0) normal (0, 1, 0) x (-1, 0, 0)
  line L0 (-467, 120) -> (-467, 114)
  line L1 (-467, 114) -> (-502, 114)
  line L2 (-502, 114) -> (-502, 120)
  line L3 (-502, 120) -> (-508, 120)
  line L4 (-508, 120) -> (-508, 114)
  line L5 (-508, 114) -> (-543, 114)
  line L6 (-543, 114) -> (-543, 120)
  line L7 (-543, 120) -> (-549, 120)
  line L8 (-549, 120) -> (-549, 114)
  line L9 (-549, 114) -> (-594, 114)
  line L10 (-594, 114) -> (-594, 99)
  line L11 (-594, 99) -> (-600, 99)
  line L12 (-600, 99) -> (-600, 93)
  line L13 (-600, 93) -> (-594, 93)
  line L14 (-594, 93) -> (-594, 73)
  line L15 (-594, 73) -> (-600, 73)
  line L16 (-600, 73) -> (-600, 67)
  line L17 (-600, 67) -> (-594, 67)
  line L18 (-594, 67) -> (-594, 47)
  line L19 (-594, 47) -> (-600, 47)
  line L20 (-600, 47) -> (-600, 41)
  line L21 (-600, 41) -> (-594, 41)
  line L22 (-594, 41) -> (-594, 26)
  line L23 (-594, 26) -> (-549, 26)
  line L24 (-549, 26) -> (-549, 20)
  line L25 (-549, 20) -> (-543, 20)
  line L26 (-543, 20) -> (-543, 26)
  line L27 (-543, 26) -> (-508, 26)
  line L28 (-508, 26) -> (-508, 20)
  line L29 (-508, 20) -> (-502, 20)
  line L30 (-502, 20) -> (-502, 26)
  line L31 (-502, 26) -> (-467, 26)
  line L32 (-467, 26) -> (-467, 20)
  line L33 (-467, 20) -> (-461, 20)
  line L34 (-461, 20) -> (-461, 26)
  line L35 (-461, 26) -> (-416, 26)
  line L36 (-416, 26) -> (-416, 41)
  line L37 (-416, 41) -> (-410, 41)
  line L38 (-410, 41) -> (-410, 47)
  line L39 (-410, 47) -> (-416, 47)
  line L40 (-416, 47) -> (-416, 67)
  line L41 (-416, 67) -> (-410, 67)
  line L42 (-410, 67) -> (-410, 73)
  line L43 (-410, 73) -> (-416, 73)
  line L44 (-416, 73) -> (-416, 93)
  line L45 (-416, 93) -> (-410, 93)
  line L46 (-410, 93) -> (-410, 99)
  line L47 (-410, 99) -> (-416, 99)
  line L48 (-416, 99) -> (-416, 114)
  line L49 (-416, 114) -> (-461, 114)
  line L50 (-461, 114) -> (-461, 120)
  line L51 (-461, 120) -> (-467, 120)
extrude "Extrude1" [suppressed]
extrude "Extrude2" [suppressed]
extrude "Extrude3" [suppressed]
extrude "Extrude4" [suppressed]
extrude "Extrude5" [suppressed]
named bodies: "frente mdf", "FRENTE", "LATERAL ESQUERDA", "LATERAL DIREITA", "FUNDO", "TOPO", "TRASEIRA", "FRENTE (1)", "TRASEIRA (1)", "LATERAL ESQUERDA (1)", "TOPO (1)", "LATERAL DIREITA (1)", "FUNDO (1)"
